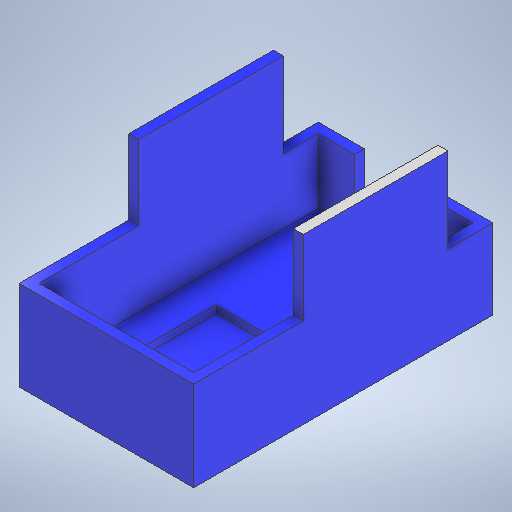
# Autodesk Inventor part: Carcaza
Saved by Autodesk Inventor 2025.1 (Build 291241020, 241B)
## iProperties
Created: 2024-08-30
Part Number: Carcaza
Material: Generic
Document SubType Name: Modeling
Designer: andre
Density: 1 g/cm^3
Appearance: Default
Author: andre
Autodesk Inventor part; units mm, degrees
ref_plane "YZ Plane" through (0, 0, 0) normal (1, 0, 0) x (0, 1, 0)
ref_plane "XZ Plane" through (0, 0, 0) normal (0, 1, 0) x (-1, 0, 0)
ref_plane "XY Plane" through (0, 0, 0) normal (0, 0, 1) x (1, 0, 0)
sketch "Sketch1" plane through (0, 0, 0) normal (0, 1, 0) x (-1, 0, 0)
  line L0 (0, 0) -> (31, 0)
  line L1 (31, 0) -> (31, -56)
  line L2 (31, -56) -> (0, -56)
  line L3 (0, -56) -> (0, 0)
  dimension "d0" = 31
  dimension "d1" = 56
  constraints: 8 end point, 2 parallel, 1 horizontal, 1 perpendicular
  measures "d0" distance of L0.start L0.end
  measures "d1" distance of L0.end L1.end
extrude "Extrusion1" add sketch "Sketch1" along normal blind 3
sketch "Sketch2" plane through (0, 3, 0) normal (0, 1, 0) x (1, 0, 0)
  line L0 (0, 56) -> (-31, 56) projected
  line L1 (-31, 56) -> (-31, 0) projected
  line L2 (-31, 0) -> (0, 0) projected
  line L3 (0, 0) -> (0, 56) projected
  line L4 (-24.5, 29) -> (-6.5, 29)
  line L5 (-6.5, 29) -> (-6.5, 10)
  line L6 (-6.5, 10) -> (-24.5, 10)
  line L7 (-24.5, 10) -> (-24.5, 29)
  line L8 (-24.5, 10) -> (-6.5, 29) construction
  line L9 (-24.5, 29) -> (-6.5, 10) construction
  line L10 (-20.25, 56) -> (-10.75, 56) construction
  line L11 (-10.75, 56) -> (-10.75, 49.5)
  line L12 (-10.75, 49.5) -> (-20.25, 49.5)
  line L13 (-20.25, 49.5) -> (-20.25, 56)
  point P0 (-15.5, 19.5)
  point P1 (-15.5, 19.5)
  point P2 (-15.5, 49.5)
  point P3 (-10.75, 52.75)
  point P4 (-15.5, 29)
  point P5 (-15.5, 10)
  point P6 (-15.5, 0)
  dimension "d4" = 18
  dimension "d5" = 19
  dimension "d8" = 6.5
  dimension "d9" = 9.5
  dimension "d32" = 39.5
  constraints: 20 end point, 7 midpoint, 4 parallel, 2 horizontal, 2 perpendicular, 2 vertical alignment, 1 point on line
  measures "d4" distance of L5.end L6.end
  measures "d5" distance of L4.end L5.end
  measures "d8" distance of L12.end L10.start
  measures "d9" distance of L11.end L12.end
  measures "d32" distance between parallel lines of L12 L6
extrude "Extrusion2" cut sketch "Sketch2" against normal blind 1.5 contours L11 L12 L13 L0 | L4 L5 L6 L7
sketch "Sketch3" plane through (0, 3, 0) normal (0, 1, 0) x (1, 0, 0)
  line L0 (-10.75, 56) -> (-10.75, 49.5) projected
  line L1 (-10.75, 49.5) -> (-20.25, 49.5) projected
  line L2 (-20.25, 49.5) -> (-20.25, 56) projected
  line L3 (-20.25, 56) -> (-31, 56) projected
  line L4 (-31, 56) -> (-31, 0) projected
  line L5 (-31, 0) -> (0, 0) projected
  line L6 (0, 0) -> (0, 56) projected
  line L7 (0, 56) -> (-10.75, 56) projected
  line L8 (-6.5, 29) -> (-6.5, 10) projected
  line L9 (-6.5, 10) -> (-24.5, 10) projected
  line L10 (-24.5, 10) -> (-24.5, 29) projected
  line L11 (-24.5, 29) -> (-6.5, 29) projected
  line L12 (-33, -2) -> (-33, 58)
  line L13 (-33, 58) -> (-23.75, 58)
  line L14 (-7.25, 58) -> (2, 58)
  line L15 (2, 58) -> (2, -2)
  line L16 (2, -2) -> (-33, -2)
  line L17 (-23.75, 58) -> (-23.75, 56)
  line L18 (-7.25, 58) -> (-7.25, 56)
  line L19 (-7.25, 58) -> (-15.5, 49.5) construction
  line L20 (-23.75, 58) -> (-15.5, 49.5) construction
  point P0 (-20.25, 58)
  point P1 (-11, 56)
  point P2 (-11, 57)
  point P3 (-20, 57)
  point P4 (-23.75, 57)
  point P5 (-25.625, 56)
  dimension "d12" = 2
  dimension "d23" = 2
  dimension "d26" = 2
  dimension "d29" = 16.5
  constraints: 18 end point, 3 midpoint, 3 point on line, 2 horizontal, 1 equal length, 1 horizontal alignment, 1 parallel, 1 vertical, 1 vertical alignment, 1 other
  measures "d12" distance between parallel lines of L4 L12
  measures "d23" distance between parallel lines of L15 L6
  measures "d26" distance from line of point (-25.625, 56) L13
  measures "d29" distance of L14.start L13.end
extrude "Extrusion3" add sketch "Sketch3" along normal blind 30 and the other way blind 3 contours L18 L14 L15 L16 L12 L13 L17 L3 L4 L5 L6 L7
sketch "Sketch4" plane through (0, 33, 0) normal (0, 1, 0) x (1, 0, 0)
  line L0 (-23.75, 58) -> (-33, 58) projected
  line L1 (-33, 58) -> (-33, -2) projected
  line L2 (-33, -2) -> (2, -2) projected
  line L3 (2, -2) -> (2, 58) projected
  line L4 (2, 58) -> (-7.25, 58) projected
  line L5 (-7.25, 56) -> (0, 56) projected
  line L6 (0, 56) -> (0, 0) projected
  line L7 (0, 0) -> (-31, 0) projected
  line L8 (-31, 0) -> (-31, 56) projected
  line L9 (-31, 56) -> (-23.75, 56) projected
  line L10 (-33, -2) -> (2, -2)
  line L11 (2, -2) -> (2, 20)
  line L12 (2, 20) -> (-33, 20)
  line L13 (-33, 20) -> (-33, -2)
  line L14 (-23.75, 56) -> (-23.75, 58) projected
  line L15 (-7.25, 58) -> (-7.25, 56) projected
  point P0 (-33, 20)
  dimension "d17" = 22
  constraints: 8 end point, 2 parallel, 1 horizontal, 1 perpendicular, 1 point on line
  measures "d17" distance between parallel lines of L2 L12
extrude "Extrusion4" cut sketch "Sketch4" against normal blind 15 contours L12 L8 L7 L6 L3 L2 L1 | L12 L6 L7 L8
sketch "Sketch6" plane through (0, 33, 0) normal (0, 1, 0) x (1, 0, 0)
  line L0 (-7.25, 58) -> (2, 58) projected
  line L1 (2, 58) -> (-33, 58)
  line L2 (-33, 58) -> (-33, 49)
  line L3 (-33, 49) -> (2, 49)
  line L4 (2, 49) -> (2, 58)
  point P0 (0, 0)
  point P1 (-11, 58)
  point P2 (-11, 58.8284)
  point P3 (-11, 58)
  point P4 (-9, 58)
  point P5 (-8, 58)
  point P6 (-5.25, 58)
  dimension "d20" = 9
  constraints: 8 end point, 2 parallel, 1 coincident, 1 horizontal, 1 perpendicular
  measures "d20" distance of L1.end L2.end
extrude "Extrusion5" cut sketch "Sketch6" against normal blind 17
sketch "Sketch8" plane through (0, 3, 0) normal (0, 1, 0) x (1, 0, 0)
  point P0 (0, 0)
sketch "Sketch7" plane through (0, 33, 0) normal (0, 1, 0) x (1, 0, 0)
  line L0 (-44.8678, -15.9016) -> (10.8124, -15.9016)
  line L1 (10.8124, -15.9016) -> (10.8124, 73.1867)
  line L2 (10.8124, 73.1867) -> (-44.8678, 73.1867)
  line L3 (-44.8678, 73.1867) -> (-44.8678, -15.9016)
  point P0 (0, 0)
  constraints: 8 end point, 2 parallel, 1 horizontal, 1 perpendicular
equation "\"d12\" = w"
equation "\"d23\" = w"
equation "\"d26\" = w"
equation "\"w\" = 2"
body "Solid1"
